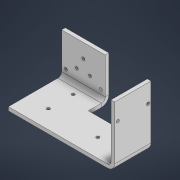
# Autodesk Inventor part: motorHolder_flipped
Saved by Autodesk Inventor 2021 (Build 250183000, 183)
## iProperties
Created: 2021-06-20
Part Number: motorHolder_flipped
Material: Generic
Document SubType Name: Sheet Metal
Designer: Watchdog
Density: 1 g/cm^3
Sheet Metal Rule: Default
Appearance: Default
Author: Watchdog
Autodesk Inventor part; units mm, degrees
ref_plane "YZ Plane" through (0, 0, 0) normal (1, 0, 0) x (0, 1, 0)
ref_plane "XZ Plane" through (0, 0, 0) normal (0, 1, 0) x (-1, 0, 0)
sketch "Sketch1" plane through (0, 0, 0) normal (0, 0, 1) x (1, 0, 0)
  line L0 (-36, 36) -> (36, 36)
  line L1 (36, 36) -> (36, -36)
  line L2 (36, -36) -> (-36, -36)
  line L3 (-36, -36) -> (-36, 36)
  point P0 (0, 0)
  dimension "d0" = 72
  dimension "d1" = 36
  dimension "d2" = 72
  dimension "d3" = 36
  measures "d0" distance between parallel lines of L2 L0
  measures "d1" distance from line of point (0, 0) L0
  measures "d2" distance between parallel lines of L1 L3
  measures "d3" distance from line of point (0, 0) L3
extrude "Plate1" add sketch "Sketch1" along normal blind 6
sketch "Sketch2" plane through (-36, -30, 6) normal (0, -1, 0) x (1, 0, 0)
  line L0 (72, 0) -> (0, 0)
  line L1 (0, 0) -> (0, -94)
  line L2 (0, -94) -> (72, -94)
  line L3 (72, -94) -> (72, 0)
  constraints: 6 end point, 1 horizontal, 1 perpendicular, 1 vertical
edge flange "Flange1" height 94 angle 90 thickness 6 bend radius 6 thickness toward (0, -1, 0) relief tear relief width 6 relief depth 3 edges at (0, -36, 0) wall of the first edge with corners at (36, -30, 6) (-36, -30, 6) (-36, -30, -88) (36, -30, -88)
bend "Bend1"
corner "Corner1"
sketch "Sketch3" plane through (-36, -30, -88) normal (0, 1, 0) x (1, 0, 0)
  line L0 (72, -82) -> (72, 0)
  line L1 (72, 0) -> (175.7, 0)
  line L2 (175.7, 0) -> (175.7, -60)
  line L3 (175.7, -60) -> (72, -60)
  line L4 (72, -60) -> (72, 0)
  point P0 (36, -88)
  dimension "d15" = 103.7
  dimension "d16" = 60
  measures "d15" distance of L2.end L3.end
  measures "d16" distance of L1.end L2.end
sheet face with bend "Face2" sketch "Sketch3" thickness 6 toward (0, -1, 0) bend radius 6
bend "Bend2"
sketch "Sketch4" plane through (133.7, -36, -88) normal (1, 0, 0) x (0, 1, 0)
  line L0 (0, 60) -> (0, 0)
  line L1 (0, 0) -> (100.6, 0)
  line L2 (100.6, 0) -> (100.6, 60)
  line L3 (100.6, 60) -> (0, 60)
  constraints: 6 end point, 1 horizontal, 1 perpendicular, 1 vertical
edge flange "Flange2" height 100.6 angle 90 thickness 6 bend radius 6 thickness toward (1, 0, 0) relief tear relief width 6 relief depth 3 edges at (139.7, -30, -58) wall of the first edge with corners at (133.7, -36, -28) (133.7, -36, -88) (133.7, 64.6, -88) (133.7, 64.6, -28)
bend "Bend3"
corner "Corner2"
sketch "Sketch5" plane through (139.7, 64.6, -28) normal (1, 0, 0) x (0, 0, -1)
  circle A0 centre (30, -30) radius 25
  line L0 (60, 0) -> (60, -88.6) projected
  line L1 (0, -88.6) -> (0, 0) projected
  line L2 (0, 0) -> (60, 0) projected
  point P0 (-28, -64.6)
  point P1 (55, -30)
  point P2 (5, -30)
  dimension "d32" = 60
  dimension "d33" = 30
  dimension "d34" = 30
  dimension "d35" = 50
  dimension "d36" = 30
  dimension "d37" = 30
  constraints: 2 point on circle, 1 centre point
  measures "d32" distance between parallel lines of L0 L1
  measures "d33" distance from line of A0.centre L1
  measures "d34" distance from line of L2 A0.centre
  measures "d35" diameter of A0
  measures "d36" distance from line of L2 A0.start
  measures "d37" distance from line of L2 A0.end
hole "Hole1" at (139.7, 34.6, -33) at (139.7, 34.6, -83) direction (-1, 0, 0) diameter 5 end through all
sketch "Sketch6" plane through (0, 0, 6) normal (0, 0, 1) x (1, 0, 0)
  circle A0 centre (0, 0) radius 12.7
  line L0 (36, -36) -> (-36, -36) projected
  circle A1 centre (0, 0) radius 33.5
  line L1 (0, 0) -> (29.0119, -16.75)
  line L2 (0, 0) -> (-29.0119, -16.75)
  line L3 (0, 0) -> (0, 33.5)
  point P0 (0, 0)
  point P1 (0, 12.7)
  point P2 (10.9985, -6.35)
  point P3 (-10.9985, -6.35)
  dimension "d45" = 36
  dimension "d46" = 25.4
  dimension "d47" = 67
  dimension "d48" = 120
  dimension "d49" = 120
  dimension "d50" = 0
  constraints: 6 end point, 6 point on circle, 3 point on line, 2 centre point, 1 coincident, 1 vertical
  measures "d45" distance from line of A0.centre L0
  measures "d46" diameter of A0
  measures "d47" diameter of A1
  measures "d48" angle of L1 L3
  measures "d49" angle of L1 L2
  measures "d50" distance of point (0, 0) A0.centre
hole "Hole2" at (0, 12.7, 6) at (-10.9985, -6.35, 6) at (10.9985, -6.35, 6) at (29.0119, -16.75, 6) at (-29.0119, -16.75, 6) direction (0, 0, -1) diameter 5 end through all
sketch "Sketch7" plane through (-36, -30, -6) normal (0, 1, 0) x (1, 0, 0)
  line L0 (163.7, 82) -> (0, 82) projected
  line L1 (163.7, 22) -> (72, 22) projected
  line L2 (0, 0) -> (0, 82) projected
  line L3 (72, 0) -> (72, 22) projected
  point P0 (36, -6)
  point P1 (117.85, 52)
  point P2 (36, 52)
  point P3 (36, 11)
  dimension "d65" = 60
  dimension "d66" = 72
  dimension "d67" = 30
  dimension "d68" = 30
  dimension "d69" = 36
  dimension "d70" = 22
  dimension "d71" = 11
  dimension "d72" = 36
  dimension "d73" = 91.7
  dimension "d74" = 45.85
  measures "d65" distance between parallel lines of L0 L1
  measures "d66" distance between parallel lines of L2 L3
  measures "d67" distance from line of L1 point (117.85, 52)
  measures "d68" distance from line of L0 point (36, 52)
  measures "d69" distance from line of L3 point (36, 11)
  measures "d70" distance of L3.start L1.end
  measures "d71" vertical distance of L1.end point (36, 11)
  measures "d72" horizontal distance of L1.end point (36, 52)
  measures "d73" distance of L1.start L1.end
  measures "d74" horizontal distance of L1.end point (117.85, 52)
hole "Hole3" at (81.85, -30, -58) at (0, -30, -58) at (0, -30, -17) direction (0, -1, 0) diameter 5 end through all
mirror "Mirror1" about plane through (133.7, -24, -88) normal (0, 0, -1)
ref_plane "Work Plane1" through (127.7, -30, -88) normal (0, 0, -1) x (-1, 0, 0)
split "Split1" plane through (127.7, -30, -88) removes the side toward (0, 0, 1)
equation "\"d67\" = 0.5 * d65"
equation "\"d68\" = 0.5 * d65"
equation "\"d69\" = 0.5 * d66"
equation "\"d71\" = 0.5 * d70"
equation "\"d72\" = 0.5 * d66"
equation "\"d74\" = 0.5 * d73"
equation "\"d1\" = 0.5 * d0"
equation "\"d2\" = d0"
equation "\"d33\" = 0.5 * d32"
equation "\"d34\" = d33"
equation "\"d36\" = d34"
equation "\"d37\" = d36"
equation "\"d43\" = Thickness"
equation "\"d49\" = d48"
equation "\"d56\" = Thickness"
equation "\"d63\" = Thickness"
equation "\"d4\" = Thickness"
equation "\"d5\" = BendReliefWidth"
equation "\"d6\" = BendReliefDepth"
equation "\"d7\" = MinimumRemnant"
equation "\"d8\" = TransitionRadius"
equation "\"d11\" = BendRadius"
equation "\"d12\" = CornerReliefSize"
equation "\"d13\" = GapSize"
equation "\"d14\" = JacobiRadiusSize"
equation "\"d17\" = BendRadius"
equation "\"d18\" = BendReliefWidth"
equation "\"d20\" = MinimumRemnant"
equation "\"d19\" = BendReliefDepth"
equation "\"d21\" = TransitionRadius"
equation "\"d22\" = BendReliefWidth"
equation "\"d23\" = BendReliefDepth"
equation "\"d24\" = MinimumRemnant"
equation "\"d25\" = TransitionRadius"
equation "\"d28\" = BendRadius"
equation "\"d29\" = CornerReliefSize"
equation "\"d30\" = GapSize"
equation "\"d31\" = JacobiRadiusSize"
equation "\"d3\" = d1"
equation "\"BendRadius\" = Thickness"
equation "\"BendReliefWidth\" = Thickness"
equation "\"BendReliefDepth\" = 0.5 * Thickness"
equation "\"CornerReliefSize\" = 4 * Thickness"
equation "\"MinimumRemnant\" = 2 * Thickness"
equation "\"TransitionRadius\" = BendRadius"
equation "\"JacobiRadiusSize\" = BendRadius"
equation "\"GapSize\" = Thickness"
equation "\"Thickness\" = 6"
body "Solid1"
